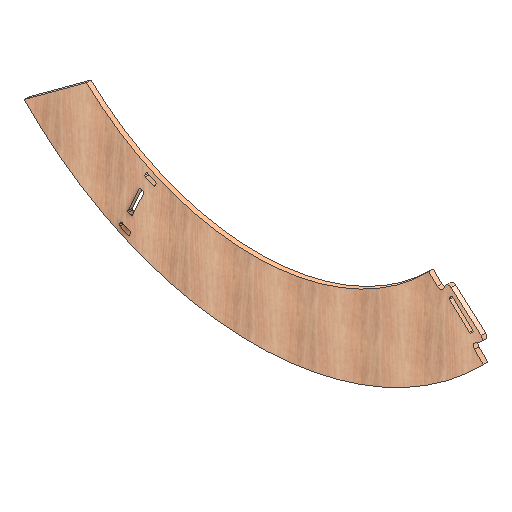
# Autodesk Inventor part: Platform D1
Saved by Autodesk Inventor 2021 (Build 250183000, 183)
## iProperties
Created: 2020-05-09
Part Number: Platform D1
Material: Wood (Birch)
Document SubType Name: Modeling
Designer: Dan Wikman
Density: 0.55 g/cm^3
Appearance: Birch - Natural Polished
Mass: 5378.64 g
Surface Area: 11772 cm^2
Volume: 9779.34 cm^3
Autodesk Inventor part; units mm, degrees
ref_plane "YZ Plane" through (0, 0, 0) normal (1, 0, 0) x (0, 1, 0)
ref_plane "XZ Plane" through (0, 0, 0) normal (0, 1, 0) x (-1, 0, 0)
ref_plane "XY Plane" through (0, 0, 0) normal (0, 0, 1) x (1, 0, 0)
sketch "CONTOURS" plane through (0, 0, 0) normal (0, 0, 1) x (1, 0, 0)
  arc A0 (1666.9081, 1038.1557) -> (1691.4363, 1042.062) centre (1677.7135, 1049.2684) ccw
  line L0 (1691.4363, 1042.062) -> (1699.2902, 1057.0177)
  arc A1 (1721.6776, 1061.1873) -> (1699.2902, 1057.0177) centre (1712.1278, 1050.2762) ccw
  line L1 (1721.6776, 1061.1873) -> (1841.3986, 956.4017)
  arc A2 (1839.5956, 933.2336) -> (1841.3986, 956.4017) centre (1831.8487, 945.4907) ccw
  line L2 (1839.5956, 933.2336) -> (1816.9578, 918.9257)
  line L3 (1814.4335, 894.7106) -> (1850.0806, 860.0494)
  arc A3 (22.5497, 860.0494) -> (1850.0806, 860.0494) centre (936.3152, 1749.5593) ccw
  line L4 (22.5497, 860.0494) -> (270.4859, 1042.1379)
  arc A4 (270.4859, 1042.1379) -> (1632.304, 1071.8026) centre (936.3091, 1749.5157) ccw
  line L5 (1632.304, 1071.8026) -> (1666.9081, 1038.1557)
  arc A5 (1816.9578, 918.9257) -> (1814.4335, 894.7106) centre (1825.2389, 905.8233) ccw
  dimension "d1" = 1275.2235
  dimension "d3" = 971.4442
  constraints: 12 end point, 12 point on circle, 6 centre point
  measures "d1" radius of A3
  measures "d3" radius of A4
sketch "HOLES" plane through (0, 0, 0) normal (0, 0, 1) x (1, 0, 0)
  line L0 (1808.3556, 951.863) -> (1800.895, 943.7797)
  arc A0 (1795.2427, 943.5532) -> (1800.895, 943.7797) centre (1797.9556, 946.4926) ccw
  line L1 (1795.2427, 943.5532) -> (1715.1445, 1017.4807)
  arc A1 (1714.9181, 1023.1331) -> (1715.1445, 1017.4807) centre (1717.8574, 1020.4201) ccw
  line L2 (1714.9181, 1023.1331) -> (1722.3786, 1031.2164)
  arc A2 (1728.031, 1031.4428) -> (1722.3786, 1031.2164) centre (1725.318, 1028.5034) ccw
  line L3 (1728.031, 1031.4428) -> (1808.1291, 957.5153)
  arc A3 (1808.3556, 951.863) -> (1808.1291, 957.5153) centre (1805.4162, 954.5759) ccw
  line L4 (543.0858, 821.5545) -> (547.6833, 831.5476)
  arc A4 (547.6833, 831.5476) -> (545.7213, 836.8533) centre (544.0494, 833.2195) ccw
  line L5 (545.7213, 836.8533) -> (513.0165, 851.8999)
  arc A5 (513.0165, 851.8999) -> (507.7108, 849.9379) centre (511.3447, 848.266) ccw
  line L6 (507.7108, 849.9379) -> (503.1133, 839.9447)
  arc A6 (503.1133, 839.9447) -> (505.0753, 834.639) centre (506.7471, 838.2729) ccw
  line L7 (505.0753, 834.639) -> (537.7801, 819.5925)
  arc A7 (537.7801, 819.5925) -> (543.0858, 821.5545) centre (539.4519, 823.2264) ccw
  line L8 (481.0423, 782.4016) -> (435.4847, 683.3788)
  arc A8 (435.4847, 683.3788) -> (437.4468, 678.0731) centre (439.1186, 681.7069) ccw
  line L9 (437.4468, 678.0731) -> (447.4399, 673.4755)
  arc A9 (447.4399, 673.4755) -> (452.7456, 675.4376) centre (449.1117, 677.1094) ccw
  line L10 (452.7456, 675.4376) -> (498.3031, 774.4603)
  arc A10 (498.3031, 774.4603) -> (496.3411, 779.766) centre (494.6693, 776.1322) ccw
  line L11 (496.3411, 779.766) -> (486.348, 784.3636)
  arc A11 (486.348, 784.3636) -> (481.0423, 782.4016) centre (484.6762, 780.7297) ccw
  line L12 (446.1185, 610.7891) -> (441.521, 600.7959)
  arc A12 (436.2153, 598.8339) -> (441.521, 600.7959) centre (437.8871, 602.4678) ccw
  line L13 (436.2153, 598.8339) -> (403.5105, 613.8804)
  arc A13 (401.5485, 619.1861) -> (403.5105, 613.8804) centre (405.1824, 617.5143) ccw
  line L14 (401.5485, 619.1861) -> (406.1461, 629.1793)
  arc A14 (411.4518, 631.1413) -> (406.1461, 629.1793) centre (409.7799, 627.5074) ccw
  line L15 (411.4518, 631.1413) -> (444.1565, 616.0948)
  arc A15 (446.1185, 610.7891) -> (444.1565, 616.0948) centre (442.4847, 612.4609) ccw
  constraints: 32 end point, 32 point on circle, 16 centre point
sketch "LETTERS" plane through (0, 0, 0) normal (0, 0, 1) x (1, 0, 0)
  line L0 (578.69, 694.1928) -> (578.8133, 694.0526)
  line L1 (578.8133, 694.0526) -> (578.9339, 693.9068)
  line L2 (578.9339, 693.9068) -> (579.0516, 693.7555)
  line L3 (579.0516, 693.7555) -> (579.1661, 693.5988)
  line L4 (579.1661, 693.5988) -> (579.2775, 693.4368)
  line L5 (579.2775, 693.4368) -> (579.3854, 693.2696)
  line L6 (579.3854, 693.2696) -> (579.4899, 693.0974)
  line L7 (579.4899, 693.0974) -> (579.5907, 692.9201)
  line L8 (579.5907, 692.9201) -> (579.6877, 692.7381)
  line L9 (579.6877, 692.7381) -> (579.7809, 692.5514)
  line L10 (579.7809, 692.5514) -> (579.87, 692.3601)
  line L11 (579.87, 692.3601) -> (579.955, 692.1646)
  line L12 (579.955, 692.1646) -> (580.0358, 691.9649)
  line L13 (580.0358, 691.9649) -> (580.1123, 691.7612)
  line L14 (580.1123, 691.7612) -> (580.1844, 691.5538)
  line L15 (580.1844, 691.5538) -> (580.252, 691.3428)
  line L16 (580.252, 691.3428) -> (580.3151, 691.1284)
  line L17 (580.3151, 691.1284) -> (580.3736, 690.911)
  line L18 (580.3736, 690.911) -> (580.4275, 690.6906)
  line L19 (580.4275, 690.6906) -> (580.4767, 690.4676)
  line L20 (580.4767, 690.4676) -> (580.5212, 690.2422)
  line L21 (580.5212, 690.2422) -> (580.561, 690.0145)
  line L22 (580.561, 690.0145) -> (580.596, 689.7849)
  line L23 (580.596, 689.7849) -> (580.6263, 689.5536)
  line L24 (580.6263, 689.5536) -> (580.6519, 689.3209)
  line L25 (580.6519, 689.3209) -> (580.6728, 689.0869)
  line L26 (580.6728, 689.0869) -> (580.689, 688.8519)
  line L27 (580.689, 688.8519) -> (580.7006, 688.6162)
  line L28 (580.7006, 688.6162) -> (580.7076, 688.3799)
  line L29 (580.7076, 688.3799) -> (580.71, 688.1435)
  line L30 (580.71, 688.1435) -> (580.7083, 687.9072)
  line L31 (580.7083, 687.9072) -> (580.7019, 687.6709)
  line L32 (580.7019, 687.6709) -> (580.6911, 687.4349)
  line L33 (580.6911, 687.4349) -> (580.6761, 687.1997)
  line L34 (580.6761, 687.1997) -> (580.6569, 686.9652)
  line L35 (580.6569, 686.9652) -> (580.6064, 686.4997)
  line L36 (580.6064, 686.4997) -> (580.5405, 686.0398)
  line L37 (580.5405, 686.0398) -> (580.46, 685.5872)
  line L38 (580.46, 685.5872) -> (580.3659, 685.1429)
  line L39 (580.3659, 685.1429) -> (580.259, 684.7083)
  line L40 (580.259, 684.7083) -> (580.1405, 684.2843)
  line L41 (580.1405, 684.2843) -> (580.0089, 683.8641)
  line L42 (580.0089, 683.8641) -> (579.8616, 683.4415)
  line L43 (579.8616, 683.4415) -> (579.6986, 683.0176)
  line L44 (579.6986, 683.0176) -> (579.5194, 682.5942)
  line L45 (579.5194, 682.5942) -> (579.3242, 682.1727)
  line L46 (579.3242, 682.1727) -> (579.1129, 681.7548)
  line L47 (579.1129, 681.7548) -> (579.0013, 681.5478)
  line L48 (579.0013, 681.5478) -> (578.8857, 681.3423)
  line L49 (578.8857, 681.3423) -> (578.7662, 681.1386)
  line L50 (578.7662, 681.1386) -> (578.6428, 680.9369)
  line L51 (578.6428, 680.9369) -> (578.5156, 680.7375)
  line L52 (578.5156, 680.7375) -> (578.3847, 680.5405)
  line L53 (578.3847, 680.5405) -> (578.2502, 680.3462)
  line L54 (578.2502, 680.3462) -> (578.1121, 680.1549)
  line L55 (578.1121, 680.1549) -> (577.9704, 679.9667)
  line L56 (577.9704, 679.9667) -> (577.8254, 679.7818)
  line L57 (577.8254, 679.7818) -> (577.6772, 679.6006)
  line L58 (577.6772, 679.6006) -> (577.5257, 679.4231)
  line L59 (577.5257, 679.4231) -> (577.3713, 679.2497)
  line L60 (577.3713, 679.2497) -> (577.2139, 679.0805)
  line L61 (577.2139, 679.0805) -> (577.0538, 678.9157)
  line L62 (577.0538, 678.9157) -> (576.891, 678.7555)
  line L63 (576.891, 678.7555) -> (576.7258, 678.6)
  line L64 (576.7258, 678.6) -> (576.5582, 678.4496)
  line L65 (576.5582, 678.4496) -> (576.3886, 678.3042)
  line L66 (576.3886, 678.3042) -> (576.2169, 678.1641)
  line L67 (576.2169, 678.1641) -> (576.0434, 678.0295)
  line L68 (576.0434, 678.0295) -> (575.8683, 677.9003)
  line L69 (575.8683, 677.9003) -> (575.6918, 677.7769)
  line L70 (575.6918, 677.7769) -> (575.5139, 677.6592)
  line L71 (575.5139, 677.6592) -> (575.335, 677.5474)
  line L72 (575.335, 677.5474) -> (575.1552, 677.4416)
  line L73 (575.1552, 677.4416) -> (574.9746, 677.3418)
  line L74 (574.9746, 677.3418) -> (574.7935, 677.2481)
  line L75 (574.7935, 677.2481) -> (574.612, 677.1606)
  line L76 (574.612, 677.1606) -> (574.4304, 677.0792)
  line L77 (574.4304, 677.0792) -> (574.2488, 677.004)
  line L78 (574.2488, 677.004) -> (574.0674, 676.9351)
  line L79 (574.0674, 676.9351) -> (573.8863, 676.8723)
  line L80 (573.8863, 676.8723) -> (573.7057, 676.8158)
  line L81 (573.7057, 676.8158) -> (573.5259, 676.7654)
  line L82 (573.5259, 676.7654) -> (573.3469, 676.7211)
  line L83 (573.3469, 676.7211) -> (573.1689, 676.6829)
  line L84 (573.1689, 676.6829) -> (572.9922, 676.6507)
  line L85 (572.9922, 676.6507) -> (572.8167, 676.6245)
  line L86 (572.8167, 676.6245) -> (572.6427, 676.6042)
  line L87 (572.6427, 676.6042) -> (572.4703, 676.5896)
  line L88 (572.4703, 676.5896) -> (572.2997, 676.5808)
  line L89 (572.2997, 676.5808) -> (572.1309, 676.5775)
  line L90 (572.1309, 676.5775) -> (571.964, 676.5797)
  line L91 (571.964, 676.5797) -> (571.7993, 676.5872)
  line L92 (571.7993, 676.5872) -> (571.6367, 676.6)
  line L93 (571.6367, 676.6) -> (571.4764, 676.6179)
  line L94 (571.4764, 676.6179) -> (571.3185, 676.6407)
  line L95 (571.3185, 676.6407) -> (571.163, 676.6683)
  line L96 (571.163, 676.6683) -> (571.0101, 676.7007)
  line L97 (571.0101, 676.7007) -> (570.8598, 676.7375)
  line L98 (570.8598, 676.7375) -> (570.7121, 676.7787)
  line L99 (578.4356, 694.4565) -> (578.564, 694.3275)
  line L100 (578.3049, 694.5797) -> (578.4356, 694.4565)
  line L101 (578.172, 694.6973) -> (578.3049, 694.5797)
  line L102 (578.0372, 694.8092) -> (578.172, 694.6973)
  line L103 (577.9006, 694.9153) -> (578.0372, 694.8092)
  line L104 (577.7623, 695.0157) -> (577.9006, 694.9153)
  line L105 (577.6225, 695.1104) -> (577.7623, 695.0157)
  line L106 (577.4814, 695.1995) -> (577.6225, 695.1104)
  line L107 (577.3392, 695.2829) -> (577.4814, 695.1995)
  line L108 (577.1959, 695.3608) -> (577.3392, 695.2829)
  line L109 (577.0518, 695.4331) -> (577.1959, 695.3608)
  line L110 (576.9069, 695.5) -> (577.0518, 695.4331)
  line L111 (576.7615, 695.5616) -> (576.9069, 695.5)
  line L112 (576.6156, 695.6178) -> (576.7615, 695.5616)
  line L113 (576.4695, 695.6688) -> (576.6156, 695.6178)
  line L114 (576.3232, 695.7147) -> (576.4695, 695.6688)
  line L115 (569.8928, 698.0178) -> (576.3232, 695.7147)
  line L116 (563.2082, 679.3542) -> (569.8928, 698.0178)
  line L117 (570.7121, 676.7787) -> (563.2082, 679.3542)
  line L118 (578.564, 694.3275) -> (578.69, 694.1928)
  constraints: 238 end point, 3 perpendicular
extrude "Extrusion2" add sketch "CONTOURS" along normal blind 18
extrude "Extrusion3" cut sketch "HOLES" along normal blind 18
body "Solid2"
